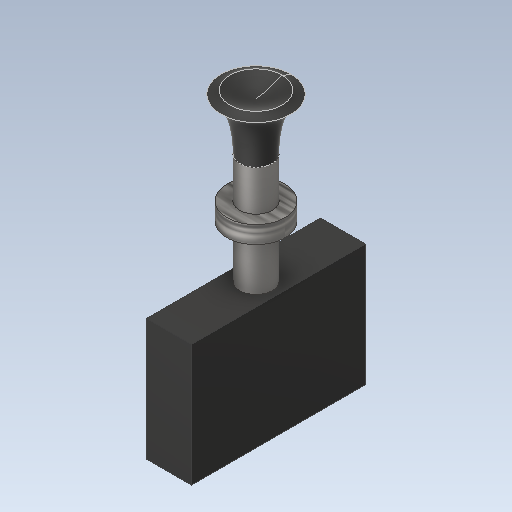
# Autodesk Inventor part: dragswitch
Saved by Autodesk Inventor 2021 (Build 250183000, 183)
## iProperties
Created: 2020-05-18
Part Number: dragswitch
Material: Generic
Document SubType Name: Modeling
Designer: Johansson
Density: 1 g/cm^3
Appearance: Default
Author: Johansson
Autodesk Inventor part; units mm, degrees
ref_plane "YZ Plane" through (0, 0, 0) normal (1, 0, 0) x (0, 1, 0)
ref_plane "XZ Plane" through (0, 0, 0) normal (0, 1, 0) x (-1, 0, 0)
sketch "Sketch1" plane through (0, 0, 0) normal (0, 1, 0) x (-1, 0, 0)
  circle A0 centre (0, 0) radius 2.8122
  constraints: 1 centre point, 1 coincident
extrude "Extrusion1" add sketch "Sketch1" along normal blind 19
sketch "Sketch2" plane through (0, 0, 0) normal (1, 0, 0) x (0, 1, 0)
  spline S0 degree 2 poles (19, -2.8122) (26.5342, -2.9696) (27.9304, -6) knots 0 0 0 1 1 1
  spline S1 degree 2 poles (27.9304, -6) (28.1632, -5.1392) (28.5405, -4.4868) knots 0 0 0 1 1 1
  spline S2 degree 2 poles (28.5405, -4.4868) (27.299, -1.7016) (27.3119, 0) knots 0 0 0 1 1 1
  line L0 (-5.7153, 0) -> (34.2916, 0) projected
  line L1 (19, 2.8122) -> (19, -2.8122) construction
  line L2 (19, -2.8122) -> (19, 2.8122) projected
  line L3 (19, -2.8122) -> (19, 0)
  line L4 (19, 0) -> (27.3119, 0)
  point P0 (0, 0)
  point P1 (25.9548, -4.0972)
  point P2 (28.2123, -5.1594)
  point P3 (27.5285, -1.6463)
  dimension "d2" = 6
  constraints: 6 end point, 2 symmetric about line, 1 midpoint, 1 perpendicular, 1 point on line, 9 other
  measures "d2" distance from line of L0 point (27.93, -6)
revolve "Revolution1" add sketch "Sketch2" angle 360 about axis through (0, -10, 0) along (0, 1, 0) separate body
sketch "Sketch3" plane through (0, 0, 0) normal (1, 0, 0) x (0, 1, 0)
  line L0 (-21, 15) -> (0, 15)
  line L1 (0, 15) -> (0, -15)
  line L2 (0, -15) -> (-21, -15)
  line L3 (-21, -15) -> (-21, 15)
  line L4 (-21, 15) -> (0, -15) construction
  line L5 (0, 15) -> (-21, -15) construction
  line L6 (-25.2, 0) -> (4.2, 0) projected
  point P0 (0, 0)
  point P1 (-10.5, 0)
  point P2 (-10.5, 0)
  dimension "d4" = 30
  dimension "d5" = 21
  constraints: 12 end point, 5 midpoint, 2 parallel, 1 horizontal, 1 perpendicular
  measures "d4" distance of L0.end L1.end
  measures "d5" distance between parallel lines of L3 L1
extrude "Extrusion2" add sketch "Sketch3" along normal mid plane 7.75 separate body
ref_plane "Work Plane1" through (-3.875, 9, 15) normal (0, 1, 0) x (1, 0, 0)
sketch "Sketch4" plane through (-3.875, 9, 15) normal (0, 1, 0) x (1, 0, 0)
  circle A0 centre (3.875, 15) radius 5
  circle A1 centre (3.875, 15) radius 2.8122 projected
  dimension "d9" = 10
  constraints: 1 centre point, 1 concentric
  measures "d9" diameter of A0
extrude "Extrusion3" add sketch "Sketch4" along normal blind 3 separate body
equation "\"d0\" = l_fastener_button"
equation "\"wl_panel\" = 285"
equation "\"t_panel\" = 8"
equation "\"r_button\" = 8"
equation "\"l_stereo\" = 178"
equation "\"d_stereo\" = 177"
equation "\"w_label\" = 15"
equation "\"r_labelscrew\" = 2.5"
equation "\"ro_labelscrew\" = 5"
equation "\"l_buttontobutton\" = 25"
equation "\"r_usboutlet\" = 29"
equation "\"l_fastener_button\" = 19"
